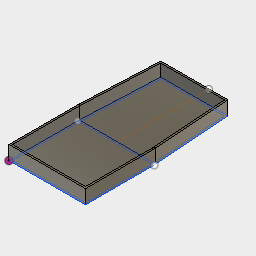
Kajütendeckel (Autodesk Fusion 360 design; units mm, degrees)
Autodesk Fusion 360 part; units mm, degrees
sketch "Sketch1" plane through (0, 0, 0) normal (0, 0, 1) x (1, 0, 0) in component "cabin_back_lid"
  line L0 (3, 3) -> (123, 3)
  line L1 (123, 3) -> (123, 113)
  line L2 (123, 113) -> (3, 113)
  line L3 (3, 113) -> (3, 3)
  line L4 (126, 0) -> (126, 116)
  line L5 (126, 116) -> (0, 116)
  line L6 (0, 116) -> (0, 0)
  line L7 (0, 0) -> (126, 0)
  line L8 (0, 116) -> (3, 113)
  line L9 (126, 116) -> (123, 113)
  line L10 (63, 116) -> (63, 266) construction
  line L11 (8.8003, 241) -> (113.8003, 241)
  line L12 (3, 113) -> (8.8003, 241)
  line L13 (123, 113) -> (113.8003, 241)
  line L14 (0.0031, 113.1358) -> (5.9332, 244)
  line L15 (5.9332, 244) -> (116.5924, 244)
  line L16 (125.9923, 113.2151) -> (116.5924, 244)
  dimension "d1" = 120
  dimension "d2" = 110
  dimension "d3" = 3
  dimension "d12" = 150
  dimension "d15" = 105
  dimension "d16" = 125
  dimension "d17" = 3
  measures "d1" distance of L0.start L0.end
  measures "d2" distance of L0.start L2.end
  measures "d12" distance of L10.start L10.end
  measures "d15" distance of L11.start L11.end
  measures "d16" distance of L5 L11
extrude "Extrude3" add sketch "Sketch1" along normal blind 23 contours L5 L8 L12 L14 | L5 L9 L13 L16 | L5 L11 L12 L13 L14 L15 L16 makes body 1 in component "cabin_back_lid"
extrude "Extrude2" add sketch "Sketch1" along normal blind 23 separate body contours L0 L1 L3 L4 L6 L7 L8 L9 makes body 2 in component "cabin_back_lid"
extrude "Extrude1" add sketch "Sketch1" along normal blind 3 separate body contours L0 L1 L2 L3 makes body 3 in component "cabin_back_lid"
extrude "Extrude4" add sketch "Sketch1" along normal blind 3 separate body contours L2 L5 L12 L13 | L5 L11 L12 L13 makes body 4 in component "cabin_back_lid"
copy_body "CutPasteBodies1" bodies 4 removing the originals makes body 5 in component "cabin_front_lid"
copy_body "CutPasteBodies2" bodies 1 removing the originals makes body 6 in component "cabin_front_lid"
component "cabin_back_lid" placed x (1, 0, 0) y (0, 1, 0) z (0, 0, 1) at (0, 0, 0)
component "cabin_front_lid" placed x (1, 0, 0) y (0, 1, 0) z (0, 0, 1) at (0, 0, 0)
equation "d1 = back_cabin_width"
equation "d2 = back_cabin_length"
equation "back_cabin_length = 110 mm"
equation "back_cabin_width = 120 mm"
equation "cabin_wall_thickness = 3 mm"
equation "cabin_lid_height = 20 mm"
equation "d8 = cabin_wall_thickness"
equation "d10 = cabin_lid_height + cabin_wall_thickness"
equation "front_cabin_length = 125 mm"
equation "front_cabin_width = 105 mm"
equation "d15 = front_cabin_width"
equation "d16 = front_cabin_length"
equation "d18 = cabin_lid_height + cabin_wall_thickness"
equation "d20 = cabin_wall_thickness"
